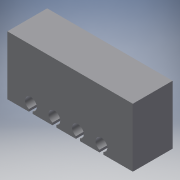
# Autodesk Inventor part: Lateral
Saved by Autodesk Inventor 2017 (Build 210142000, 142)
## iProperties
Created: 2021-02-12
Part Number: Lateral
Material: Generic
Document SubType Name: Modeling
Designer: USUARIO
Density: 1 g/cm^3
Appearance: Default
Author: USUARIO
Autodesk Inventor part; units mm, degrees
ref_plane "YZ Plane" through (0, 0, 0) normal (1, 0, 0) x (0, 1, 0)
ref_plane "XZ Plane" through (0, 0, 0) normal (0, 1, 0) x (-1, 0, 0)
ref_plane "XY Plane" through (0, 0, 0) normal (0, 0, 1) x (1, 0, 0)
sketch "Sketch1" plane through (0, 0, 0) normal (0, 1, 0) x (-1, 0, 0)
  line L0 (0, 0) -> (160, 0)
  line L1 (160, 0) -> (160, -75)
  line L2 (160, -75) -> (0, -75)
  line L3 (0, -75) -> (0, 0)
  dimension "d0" = 160
  dimension "d1" = 75
  constraints: 8 end point, 2 parallel, 1 horizontal, 1 perpendicular
  measures "d0" distance of L1.end L2.end
  measures "d1" distance of L0.end L1.end
extrude "Extrusion1" add sketch "Sketch1" along normal blind 50.8
sketch "Sketch2" plane through (0, 50.8, 0) normal (0, 1, 0) x (1, 0, 0)
  circle A0 centre (-110, 65) radius 6.5
  line L0 (0, 75) -> (-160, 75) projected
  line L1 (-160, 75) -> (-160, 0) projected
  circle A1 centre (-90, 65) radius 6.5
  circle A2 centre (-70, 65) radius 6.5
  circle A3 centre (-50, 65) radius 6.5
  point P0 (0, 0)
  dimension "d4" = 13
  dimension "d5" = 10
  dimension "d6" = 50
  dimension "d12" = 20
  constraints: 4 centre point, 1 horizontal, 6 other
  measures "d4" diameter of A0
  measures "d5" distance from line of A0.centre L0
  measures "d6" distance from line of A0.centre L1
  measures "d12" distance of A0.centre A1.centre
extrude "Extrusion2" cut sketch "Sketch2" against normal blind 50.8
sketch "Sketch3" plane through (0, 50.8, 0) normal (0, 1, 0) x (1, 0, 0)
  line L0 (0, 75) -> (-160, 75) projected
  line L1 (-112.5, 75) -> (-107.5, 75)
  line L2 (-107.5, 75) -> (-107.5, 70)
  line L3 (-107.5, 70) -> (-112.5, 70)
  line L4 (-112.5, 70) -> (-112.5, 75)
  circle A0 centre (-110, 65) radius 6.5 projected
  line L5 (-87.5, 75) -> (-87.5, 70)
  line L6 (-87.5, 70) -> (-92.5, 70)
  line L7 (-92.5, 70) -> (-92.5, 75)
  line L8 (-92.5, 75) -> (-87.5, 75)
  line L9 (-67.5, 75) -> (-67.5, 70)
  line L10 (-67.5, 70) -> (-72.5, 70)
  line L11 (-72.5, 70) -> (-72.5, 75)
  line L12 (-72.5, 75) -> (-67.5, 75)
  line L13 (-47.5, 75) -> (-47.5, 70)
  line L14 (-47.5, 70) -> (-52.5, 70)
  line L15 (-52.5, 70) -> (-52.5, 75)
  line L16 (-52.5, 75) -> (-47.5, 75)
  point P0 (0, 0)
  dimension "d16" = 5
  dimension "d17" = 5
  dimension "d18" = 2.5
  dimension "d24" = 20
  constraints: 32 end point, 2 horizontal, 2 parallel, 1 perpendicular, 1 point on line, 24 other
  measures "d16" distance of L2.end L3.end
  measures "d17" distance of L1.end L2.end
  measures "d18" distance from line of L4 A0.centre
  measures "d24" distance of L1.end L5.start
extrude "Extrusion3" cut sketch "Sketch3" against normal blind 50.8 contours L13 L14 L15 L0 | L2 A0 L4 L0 | L5 L6 L7 L0 | L9 L10 L11 L0 | L2 L3 L4 A0 picked at (-110, 70.5)
body "Solid1"
